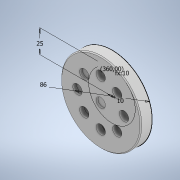
# Autodesk Inventor part: Diameter_10mm
Saved by Autodesk Inventor 2021 (Build 250183000, 183)
## iProperties
Created: 2023-09-28
Part Number: Diameter_10mm
Material: Generic
Document SubType Name: Modeling
Designer: Konstantin
Density: 1 g/cm^3
Appearance: Default
Author: Konstantin
Autodesk Inventor part; units mm, degrees
ref_plane "YZ Plane" through (0, 0, 0) normal (1, 0, 0) x (0, 1, 0)
ref_plane "XZ Plane" through (0, 0, 0) normal (0, 1, 0) x (-1, 0, 0)
ref_plane "XY Plane" through (0, 0, 0) normal (0, 0, 1) x (1, 0, 0)
sketch "Sketch1" plane through (0, 0, 0) normal (0, 0, 1) x (1, 0, 0)
  circle A0 centre (0, 0) radius 43
  circle A1 centre (0, 0) radius 5
  circle A2 centre (0, 25) radius 5
  circle A3 centre (-17.6777, 17.6777) radius 5
  circle A4 centre (-25, 0) radius 5
  circle A5 centre (-17.6777, -17.6777) radius 5
  circle A6 centre (0, -25) radius 5
  circle A7 centre (17.6777, -17.6777) radius 5
  circle A8 centre (25, 0) radius 5
  circle A9 centre (17.6777, 17.6777) radius 5
  dimension "diameter" = 10
  dimension "d2" = 10
  dimension "d5" = 360
  dimension "d7" = 25
  dimension "d28" = 86
  constraints: 10 centre point, 2 coincident, 17 other
  measures "diameter" diameter of A1
  measures "d2" diameter of A2
  measures "d7" distance of point (0, 0) A2.centre
  measures "d28" diameter of A0
extrude "Extrusion1" add sketch "Sketch1" along normal blind 12
extrude "Extrusion2" add sketch "Sketch1" along normal blind 2 contours A2
extrude "Extrusion3" add sketch "Sketch1" along normal blind 3 contours A9
extrude "Extrusion4" add sketch "Sketch1" along normal blind 4 contours A8
extrude "Extrusion5" add sketch "Sketch1" along normal blind 5 contours A7
extrude "Extrusion6" add sketch "Sketch1" along normal blind 6 contours A6
extrude "Extrusion7" add sketch "Sketch1" along normal blind 7 contours A5
extrude "Extrusion8" add sketch "Sketch1" along normal blind 8 contours A4
extrude "Extrusion9" add sketch "Sketch1" along normal blind 9 contours A3
extrude "Extrusion10" add sketch "Sketch1" along normal blind 10 contours A1
sketch "Sketch2" plane through (0, 0, 12) normal (0, 0, 1) x (1, 0, 0)
  line L0 (-5.8774, 39.105) -> (5.7366, 39.105) construction
  line L1 (5.7366, 39.105) -> (5.7366, 35.936) construction
  line L2 (5.7366, 35.936) -> (-5.8774, 35.936) construction
  line L3 (-5.8774, 35.936) -> (-5.8774, 39.105) construction
  point P0 (0, 0)
  constraints: 2 other
emboss "Emboss1" [suppressed]
chamfer "Chamfer1" distance 1 angle 45 1 edges at (-43, 0, 12)
equation "\"d2\" = diameter"
body "Solid1"
